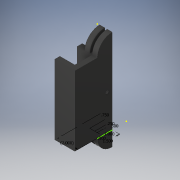
# Autodesk Inventor part: SUspension mounting
Saved by Autodesk Inventor 2018.2 (Build 222227000, 227)
## iProperties
Created: 2018-02-01
Part Number: SUspension mounting
Material: Acetal Resin, Black
Document SubType Name: Modeling
Designer: MIABo
Density: 1.425 g/cm^3
Appearance: Smooth - Black
Author: MIABo
Autodesk Inventor part; units mm, degrees
ref_plane "YZ Plane" through (0, 0, 0) normal (1, 0, 0) x (0, 1, 0)
ref_plane "XZ Plane" through (0, 0, 0) normal (0, 1, 0) x (-1, 0, 0)
ref_plane "XY Plane" through (0, 0, 0) normal (0, 0, 1) x (1, 0, 0)
sketch "Sketch1" plane through (0, 0, 0) normal (0, 1, 0) x (-1, 0, 0)
  line L0 (-43.0833, 36.6301) -> (-43.0833, 62.0301)
  line L1 (-74.8333, 74.7301) -> (-74.8333, 36.6301)
  line L2 (-74.8333, 36.6301) -> (-62.1333, 36.6301)
  line L3 (-62.1333, 36.6301) -> (-62.1333, 62.0301)
  line L4 (-62.1333, 62.0301) -> (-55.7833, 62.0301)
  line L5 (-55.7833, 62.0301) -> (-55.7833, 36.6301)
  line L6 (-55.7833, 36.6301) -> (-43.0833, 36.6301)
  line L7 (-43.0833, 62.0301) -> (-24.0333, 62.0301)
  line L8 (-24.0333, 62.0301) -> (-24.0333, 74.7301)
  line L9 (-24.0333, 74.7301) -> (-74.8333, 74.7301)
  point P0 (0, 0)
  dimension "d2" = 6.35
  dimension "d4" = 25.4
  dimension "d18" = 12.7
  dimension "d19" = 38.1
  dimension "d20" = 12.7
  dimension "d21" = 19.05
  dimension "d39" = 50.8
  constraints: 20 end point, 7 perpendicular, 1 collinear, 1 horizontal, 1 parallel, 1 point on line, 1 vertical
  measures "d2" distance of L3.end L4.end
  measures "d4" distance of L2.end L3.end
  measures "d18" distance between parallel lines of L9 L7
  measures "d19" distance of L1.start L1.end
  measures "d20" distance of L1.end L2.end
  measures "d21" distance of L0.end L7.end
  measures "d39" distance of L8.end L1.start
extrude "Extrusion1" add sketch "Sketch1" along normal blind 177.8
sketch "Sketch2" plane through (74.8333, 0, 74.7301) normal (1, 0, 0) x (0, 0, -1)
  line L0 (0, 177.8) -> (38.1, 177.8) projected
  line L1 (38.1, 0) -> (38.1, 177.8) projected
  line L2 (0, 0) -> (38.1, 0) projected
  point P0 (74.7301, 0)
  point P1 (25.4, 88.9)
  point P2 (0, 152.4)
  dimension "d8" = 88.9
  dimension "d9" = 12.7
  dimension "d32" = 177.8
  constraints: 1 other
  measures "d9" distance from line of point (25.4, 88.9) L1
hole "Hole1" at (74.8333, 88.9, 49.3301) direction (-1, 0, 0) diameter 6.35 end through all
sketch "Sketch7" plane through (0, 177.8, 0) normal (0, 1, 0) x (1, 0, 0)
  line L0 (74.8333, -74.7301) -> (74.8333, -36.6301) projected
  line L1 (74.8333, -74.7301) -> (74.8333, -36.6301)
  line L2 (74.8333, -36.6301) -> (62.1333, -36.6301) projected
  line L3 (74.8333, -36.6301) -> (62.1333, -36.6301)
  line L4 (62.1333, -62.0301) -> (55.7833, -62.0301) projected
  line L5 (62.1333, -36.6301) -> (62.1333, -62.0301)
  line L6 (55.7833, -62.0301) -> (55.7833, -36.6301)
  line L7 (55.7833, -36.6301) -> (43.0833, -36.6301) projected
  line L8 (55.7833, -36.6301) -> (43.0833, -36.6301)
  line L9 (43.0833, -36.6301) -> (43.0833, -74.7301)
  line L10 (43.0833, -74.7301) -> (55.7833, -74.7301)
  line L11 (24.0333, -74.7301) -> (74.8333, -74.7301) projected
  line L12 (62.1333, -36.6301) -> (62.1333, -62.0301) projected
  line L13 (62.1333, -62.0301) -> (62.1333, -74.7301)
  line L14 (55.7833, -62.0301) -> (55.7833, -74.7301)
  line L15 (62.1333, -62.0301) -> (62.1333, -74.7301)
  point P0 (0, 0)
  constraints: 20 end point, 5 point on line, 4 collinear, 2 perpendicular, 1 vertical
revolve "Revolution4" add sketch "Sketch7" angle 90 about axis through (55.7833, 177.8, 36.6301) along (-1, 0, 0) contours L10 L9 L7 L6 L14
sketch "Sketch8" plane through (0, 177.8, 0) normal (0, 1, 0) x (1, 0, 0)
  line L0 (74.8333, -74.7301) -> (74.8333, -36.6301) projected
  line L1 (74.8333, -74.7301) -> (74.8333, -36.6301)
  line L2 (74.8333, -36.6301) -> (62.1333, -36.6301) projected
  line L3 (74.8333, -36.6301) -> (62.1333, -36.6301)
  line L4 (62.1333, -36.6301) -> (62.1333, -74.7301)
  line L5 (24.0333, -74.7301) -> (74.8333, -74.7301) projected
  point P0 (0, 0)
  constraints: 6 end point, 1 collinear, 1 perpendicular, 1 point on line, 1 vertical
revolve "Revolution5" add sketch "Sketch8" angle 90 about axis through (74.8333, 177.8, 36.6301) along (-1, 0, 0)
sketch "Sketch9" plane through (0, 0, 0) normal (0, -1, 0) x (1, 0, 0)
  line L0 (55.7833, 36.6301) -> (43.0833, 36.6301) projected
  line L1 (43.0833, 74.7301) -> (55.7833, 74.7301)
  line L2 (55.7833, 62.0301) -> (55.7833, 36.6301)
  line L3 (55.7833, 36.6301) -> (43.0833, 36.6301)
  line L4 (55.7833, 74.7301) -> (55.7833, 36.6301) projected
  line L5 (43.0833, 36.6301) -> (55.7833, 36.6301)
  line L6 (55.7833, 36.6301) -> (55.7833, 74.7301)
  line L7 (55.7833, 74.7301) -> (43.0833, 74.7301)
  line L8 (43.0833, 74.7301) -> (43.0833, 36.6301)
  line L9 (74.8333, 36.6301) -> (62.1333, 36.6301) projected
  line L10 (62.1333, 36.6301) -> (62.1333, 74.7301)
  line L11 (24.0333, 74.7301) -> (74.8333, 74.7301) projected
  line L12 (74.8333, 74.7301) -> (74.8333, 36.6301) projected
  line L13 (74.8333, 74.7301) -> (74.8333, 36.6301)
  line L14 (62.1333, 36.6301) -> (62.1333, 62.0301) projected
  line L15 (74.8333, 36.6301) -> (62.1333, 36.6301)
  point P0 (0, 0)
  constraints: 20 end point, 3 equal length, 3 perpendicular, 1 horizontal, 1 point on line, 1 vertical
revolve "Revolution6" add sketch "Sketch9" angle 90 about axis through (74.8333, 0, 36.6301) along (1, 0, 0) contours L9 L10 L11 L12
sketch "Sketch10" plane through (0, 0, 0) normal (0, -1, 0) x (1, 0, 0)
  line L0 (43.0833, 74.7301) -> (55.7833, 74.7301) projected
  line L1 (43.0833, 36.6301) -> (43.0833, 74.7301)
  line L2 (55.7833, 74.7301) -> (55.7833, 36.6301) projected
  line L3 (43.0833, 74.7301) -> (55.7833, 74.7301)
  line L4 (55.7833, 74.7301) -> (55.7833, 36.6301)
  line L5 (55.7833, 36.6301) -> (43.0833, 36.6301) projected
  line L6 (55.7833, 36.6301) -> (43.0833, 36.6301)
  point P0 (0, 0)
  constraints: 8 end point, 2 perpendicular, 1 collinear, 1 vertical
revolve "Revolution7" add sketch "Sketch10" angle 90 about axis through (55.7833, 0, 36.6301) along (1, 0, 0)
sketch "Sketch12" plane through (74.8333, -38.1, 36.6301) normal (1, 0, 0) x (0, 0, -1)
  point P0 (36.6301, 38.1)
sketch "Sketch13" plane through (24.0333, 0, 74.7301) normal (0, 0, 1) x (1, 0, 0)
  line L0 (38.1, -38.1) -> (38.1, 215.9) projected
  line L1 (38.1, 0) -> (50.8, 0)
  line L2 (50.8, 0) -> (50.8, 178.176)
  line L3 (50.8, 178.176) -> (38.1, 178.176)
  line L4 (38.1, 178.176) -> (38.1, 0)
  point P0 (-24.0333, 0)
  dimension "d33" = 12.7
  constraints: 8 end point, 2 parallel, 1 horizontal, 1 perpendicular, 1 point on line
  measures "d33" distance between parallel lines of L2 L0
extrude "Extrusion2" add sketch "Sketch13" along normal blind 57.15
sketch "Sketch14" plane through (62.1333, 0, 74.7301) normal (-1, 0, 0) x (0, 0, 1)
  line L0 (57.15, 0) -> (57.15, 178.176) projected
  line L1 (0, 178.176) -> (57.15, 178.176) projected
  line L2 (57.15, 0) -> (44.45, 0)
  line L3 (44.45, 0) -> (44.45, 178.176)
  line L4 (44.45, 178.176) -> (57.15, 178.176)
  line L5 (57.15, 178.176) -> (57.15, 0)
  point P0 (-74.7301, 0)
  dimension "d36" = 12.7
  constraints: 8 end point, 2 parallel, 1 horizontal, 1 perpendicular, 1 point on line
  measures "d36" distance of L0.start L2.end
extrude "Extrusion3" add sketch "Sketch14" along normal blind 38.1
sketch "Sketch15" plane through (62.1333, 178.176, 74.7301) normal (0, 1, 0) x (1, 0, 0)
  point P0 (-62.1333, 74.7301)
body "Solid1"
